Autodesk Fusion 360 part; units mm, degrees
(part 3 of 3)
sketch "Sketch8" plane through (0, 0, 14) normal (0, 0, -1) x (1, 0, 0)
  line L0 (65.5351, 21) -> (80.5351, 21)
  line L1 (80.5351, 21) -> (80.5351, 35)
  line L2 (80.5351, 35) -> (65.5351, 35)
  line L3 (65.5351, 35) -> (65.5351, 21)
  line L4 (80.5351, 21) -> (65.5351, 21)
  line L5 (65.5351, 21) -> (65.5351, 7)
  line L6 (65.5351, 7) -> (80.5351, 7)
  line L7 (80.5351, 7) -> (80.5351, 21)
  line L8 (76.5351, 8) -> (69.5351, 8)
  line L9 (69.5351, 8) -> (69.5351, 34)
  line L10 (69.5351, 34) -> (76.5351, 34)
  line L11 (76.5351, 34) -> (76.5351, 8)
  line L12 (76.5351, 8) -> (69.5351, 34) construction
  line L13 (69.5351, 8) -> (76.5351, 34) construction
  line L14 (80.6351, 20.9) -> (80.6351, 35.1)
  line L15 (80.6351, 35.1) -> (65.4351, 35.1)
  line L16 (65.4351, 35.1) -> (65.4351, 20.9)
  line L17 (65.4351, 20.9) -> (80.6351, 20.9)
  line L18 (80.6351, 6.9) -> (80.6351, 21.1)
  line L19 (80.6351, 21.1) -> (65.4351, 21.1)
  line L20 (65.4351, 21.1) -> (65.4351, 6.9)
  line L21 (65.4351, 6.9) -> (80.6351, 6.9)
  line L22 (81.5351, 20) -> (81.5351, 36)
  line L23 (81.5351, 36) -> (64.5351, 36)
  line L24 (64.5351, 36) -> (64.5351, 20)
  line L25 (81.5351, 6) -> (81.5351, 22)
  line L26 (64.5351, 22) -> (64.5351, 6)
  line L27 (64.5351, 6) -> (81.5351, 6)
  line L28 (65.4351, 20) -> (65.5351, 20)
  line L29 (80.5351, 20) -> (80.6351, 20)
  line L30 (80.6351, 22) -> (80.5351, 22)
  line L31 (65.5351, 22) -> (65.4351, 22)
  point P0 (73.0351, 21)
  dimension "d278" = 7
  dimension "d279" = 26
  dimension "d280" = 0.1
  dimension "d281" = 0.1
  constraint horizontal L8
  constraint perpendicular L8 L9
  constraint parallel L8 L10
  constraint parallel L9 L11
  constraint coincident L12 P0
  constraint coincident L13 P0
  constraint midpoint L0 P0
  constraint coincident L5 L28.end
  constraint coincident L7 L29.start
  constraint coincident L18 L29.end
  constraint coincident L20 L28.start
  constraint coincident L16 L31.end
  constraint coincident L14 L30.start
  constraint coincident L1 L30.end
  constraint collinear L30 L31
  constraint coincident L3 L31.start
  measures "d278" distance of L9.end L10.end
  measures "d279" distance of L8.end L9.end
extrude "Extrude41" add sketch "Sketch8" against normal blind 8.5 from surface at 12 contours L0 L4 L9 L11 L19 | L0 L4 L9 L11 L17 | L8 L9 L11 L17 | L9 L10 L11 L19 bodies 13
fillet "Fillet7" radius 1.5 4 edges at (76.5351, -21, 10.5) (69.5351, -21, 10.5) (73.0351, -34, 10.5) (73.0351, -8, 10.5) on bodies 13
extrude "Extrude42" cut sketch "Sketch8" against normal blind 4 contours L0 L3 L4 L9 L19 | L3 L5 L16 L17 L19 L20 | L0 L4 L5 L9 L17 | L3 L16 L19 L31 | L1 L2 L3 L9 L10 L11 L19 | L5 L6 L7 L8 L9 L11 L17 | L5 L17 L20 L28 | L0 L1 L4 L11 L19 | L0 L4 L7 L11 L17 | L1 L2 L3 L14 L15 L16 L30 L31 | L5 L6 L7 L18 L20 L21 L28 L29 | L1 L7 L14 L17 L18 L19 | L1 L14 L19 L30 | L7 L17 L18 L29 | L22 L23 L24 L25 L26 L27 bodies 15
extrude "Extrude43" cut sketch "Sketch8" against normal blind 6 contours L0 L3 L4 L9 L19 | L0 L4 L5 L9 L17 | L1 L2 L3 L9 L10 L11 L19 | L5 L6 L7 L8 L9 L11 L17 | L0 L1 L4 L11 L19 | L0 L4 L7 L11 L17 bodies 12
sketch "Sketch9" plane through (0, 0, 10.5) normal (0, 0, 1) x (-1, 0, 0)
  line L0 (-71.0351, 9.5) -> (-71.0351, 32.5)
  line L1 (-71.0351, 32.5) -> (-75.0351, 32.5)
  line L2 (-75.0351, 32.5) -> (-75.0351, 9.5)
  line L3 (-75.0351, 9.5) -> (-71.0351, 9.5)
  line L4 (-71.0351, 20) -> (-75.0351, 20)
  line L5 (-75.0351, 20) -> (-75.0351, 22.4)
  line L6 (-75.0351, 22.4) -> (-71.0351, 22.4)
  line L7 (-71.0351, 22.4) -> (-71.0351, 20)
  line L8 (-75.0351, 20) -> (-71.0351, 20) construction
  line L9 (-71.0351, 20) -> (-71.0351, 12.1) construction
  line L10 (-71.0351, 12.1) -> (-75.0351, 12.1) construction
  line L11 (-75.0351, 12.1) -> (-75.0351, 20) construction
  line L12 (-75.0351, 22.4) -> (-71.0351, 22.4) construction
  line L13 (-71.0351, 22.4) -> (-71.0351, 30.3) construction
  line L14 (-71.0351, 30.3) -> (-75.0351, 30.3) construction
  line L15 (-75.0351, 30.3) -> (-75.0351, 22.4) construction
  line L16 (-75.0351, 30.3) -> (-71.0351, 30.3)
  line L17 (-71.0351, 30.3) -> (-71.0351, 32.3)
  line L18 (-71.0351, 32.3) -> (-75.0351, 32.3)
  line L19 (-75.0351, 32.3) -> (-75.0351, 30.3)
  line L20 (-75.0351, 12.1) -> (-71.0351, 12.1)
  line L21 (-71.0351, 12.1) -> (-71.0351, 10.1)
  line L22 (-71.0351, 10.1) -> (-75.0351, 10.1)
  line L23 (-75.0351, 10.1) -> (-75.0351, 12.1)
  dimension "d295" = 2.4
  dimension "d296" = 7.9
  dimension "d297" = 7.9
  dimension "d298" = 2
  dimension "d299" = 2
  constraint horizontal L4
  constraint perpendicular L4 L5
  constraint parallel L4 L6
  constraint parallel L5 L7
  constraint horizontal L8
  constraint vertical L9
  constraint horizontal L10
  constraint vertical L11
  constraint horizontal L12
  constraint vertical L13
  constraint horizontal L14
  constraint vertical L15
  constraint horizontal L16
  constraint vertical L17
  constraint horizontal L18
  constraint vertical L19
  constraint horizontal L20
  constraint vertical L21
  constraint horizontal L22
  constraint vertical L23
  measures "d295" distance of L4.end L5.end
  measures "d296" distance of L4.end L10.end
  measures "d297" distance of L5.end L14.end
  measures "d298" distance of L14.end L18.end
  measures "d299" distance of L10.end L22.end
extrude "Extrude44" add sketch "Sketch9" along normal blind 2.6 contours L0 L2 L20 L21 L22 L23 | L0 L2 L4 L5 L6 L7 | L0 L2 L16 L17 L18 L19 bodies 13
chamfer "Chamfer9" distance 1 angle 45 6 edges at (53.5294, -9.8942, 12.5) (24.8248, -9.8942, 12.5) (1.062, -9.8942, 12.5) (24.8248, -32.8942, 12.5) (42.3772, -32.8942, 12.5) (1.062, -32.8942, 12.5) on bodies 12
extrude "Extrude45" add sketch "Sketch7" along normal blind 2 from surface at 7 contours L55 L69 L73 L86 | L68 L69 L70 L73 L74 L75 L87 L88 | L55 L68 L75 L84 L85 bodies 16
sketch "Sketch10" plane through (0, 0, 0) normal (0, 0, 1) x (1, 0, 0)
  line L0 (0, -124.6556) -> (3.5, -124.6556)
  line L1 (3.5, -124.6556) -> (3.5, -128.1556)
  line L2 (3.5, -128.1556) -> (0, -128.1556)
  line L3 (0, -128.1556) -> (0, -124.6556)
  line L4 (-1, -129.1556) -> (-1, -123.6556)
  line L5 (-1, -123.6556) -> (4.5, -123.6556)
  line L6 (4.5, -123.6556) -> (4.5, -129.1556)
  line L7 (4.5, -129.1556) -> (-1, -129.1556)
  line L8 (19.9601, -130.9847) -> (33.4601, -130.9847)
  line L9 (33.4601, -130.9847) -> (33.4601, -103.5847)
  line L10 (33.4601, -103.5847) -> (19.9601, -103.5847)
  line L11 (19.9601, -103.5847) -> (19.9601, -130.9847)
  line L12 (26.7101, -130.9847) -> (26.7101, -123.1847) construction
  line L13 (19.9601, -123.1847) -> (26.5601, -123.1847) construction
  line L14 (30.4601, -119.2847) -> (22.6601, -119.2847) construction
  line L15 (22.6601, -119.2847) -> (22.6601, -127.0847) construction
  line L16 (22.6601, -127.0847) -> (30.4601, -127.0847) construction
  line L17 (30.4601, -127.0847) -> (30.4601, -119.2847) construction
  line L18 (30.4601, -119.2847) -> (22.6601, -127.0847) construction
  line L19 (22.6601, -119.2847) -> (30.4601, -127.0847) construction
  line L20 (19.9601, -130.9847) -> (22.4601, -130.9847)
  line L21 (22.4601, -130.9847) -> (22.4601, -119.2847)
  line L22 (22.4601, -119.2847) -> (19.9601, -119.2847)
  line L23 (19.9601, -119.2847) -> (19.9601, -130.9847)
  line L24 (33.4601, -130.9847) -> (30.8601, -130.9847)
  line L25 (30.8601, -130.9847) -> (30.8601, -119.2847)
  line L26 (30.8601, -119.2847) -> (33.4601, -119.2847)
  line L27 (33.4601, -119.2847) -> (33.4601, -130.9847)
  line L28 (28.2101, -127.778) -> (25.2101, -127.778)
  line L29 (25.2101, -127.778) -> (25.2101, -129.778)
  line L30 (25.2101, -129.778) -> (28.2101, -129.778)
  line L31 (28.2101, -129.778) -> (28.2101, -127.778)
  line L32 (28.2101, -127.778) -> (25.2101, -129.778) construction
  line L33 (25.2101, -127.778) -> (28.2101, -129.778) construction
  line L34 (25.2101, -129.778) -> (25.2101, -130.9847)
  line L35 (28.2101, -129.778) -> (28.2101, -130.9847)
  point P0 (26.5601, -123.1847)
  point P1 (26.7101, -128.778)
  dimension "d307" = 3.5
  dimension "d308" = 3.5
  dimension "d309" = -1
  dimension "d314" = 13.5
  dimension "d315" = 27.4
  dimension "d316" = 7.8
  dimension "d317" = 6.6
  dimension "d318" = 7.8
  dimension "d319" = 7.8
  dimension "d320" = 2.5
  dimension "d321" = 2.6
  dimension "d322" = 3
  dimension "d323" = 2
  constraint horizontal L0
  constraint vertical L1
  constraint horizontal L2
  constraint vertical L3
  constraint horizontal L8
  constraint vertical L9
  constraint horizontal L10
  constraint vertical L11
  constraint midpoint L8 L12.start
  constraint perpendicular L8 L12
  constraint coincident L11 L13.start
  constraint perpendicular L12 L13
  constraint horizontal L14
  constraint perpendicular L14 L15
  constraint parallel L14 L16
  constraint parallel L15 L17
  constraint coincident L18 P0
  constraint coincident L19 P0
  constraint coincident P0 L13.end
  constraint horizontal L20
  constraint vertical L21
  constraint horizontal L22
  constraint vertical L23
  constraint horizontal L24
  constraint vertical L25
  constraint horizontal L26
  constraint vertical L27
  constraint horizontal L28
  constraint perpendicular L28 L29
  constraint parallel L28 L30
  constraint parallel L29 L31
  constraint coincident L32 P1
  constraint coincident L33 P1
  constraint coincident L12 P1
  constraint coincident L8 L34.end
  constraint perpendicular L8 L34
  constraint coincident L8 L35.end
  constraint perpendicular L8 L35
  measures "d307" distance of L0.start L0.end
  measures "d308" distance of L0.start L2.end
  measures "d314" distance of L8.start L8.end
  measures "d315" distance of L8.start L10.end
  measures "d316" distance of L12.start L12.end
  measures "d317" distance of L13.start P0
  measures "d318" distance of L15.end L16.end
  measures "d319" distance of L14.end L15.end
  measures "d320" distance of L8.start L20.end
  measures "d321" distance of L8.end L24.end
  measures "d322" distance of L29.end L30.end
  measures "d323" distance of L28.end L29.end
extrude "Extrude46" add sketch "Sketch10" along normal blind 7.3 separate body contours L0 L1 L2 L3 makes body 19
extrude "Extrude47" add sketch "Sketch10" along normal blind 1 contours L4 L5 L6 L7 bodies 19
extrude "Extrude48" add sketch "Sketch10" against normal blind 2 separate body contours L8 L11 L20 L21 L22 L23 | L8 L9 L10 L11 L21 L22 L25 L26 L28 L29 L31 L34 L35 | L8 L30 L34 L35 | L28 L29 L30 L31 | L8 L9 L24 L25 L26 L27 makes body 20
sketch "Sketch11" plane through (0, 0, 16.5) normal (0, 0, 1) x (-1, 0, 0)
  line L0 (-80.5351, 35) -> (-65.5351, 35)
  line L1 (-65.5351, 35) -> (-65.5351, 7)
  line L2 (-65.5351, 7) -> (-80.5351, 7)
  line L3 (-80.5351, 7) -> (-80.5351, 35)
  line L4 (2, -114) -> (3, -114)
  line L5 (3, -114) -> (3, -129)
  line L6 (3, -129) -> (15, -129)
  line L7 (15, -129) -> (15, -114)
  line L8 (15, -114) -> (16, -114)
  line L9 (16, -114) -> (16, 35)
  arc A0 (16, 35) -> (6, 45) centre (6, 35) ccw
  line L10 (6, 45) -> (-84, 45)
  arc A1 (-84, 45) -> (-94, 35) centre (-84, 35) ccw
  line L11 (-94, 35) -> (-94, -114)
  line L12 (-94, -114) -> (-93, -114)
  line L13 (-93, -114) -> (-93, -129)
  line L14 (-93, -129) -> (-81, -129)
  line L15 (-81, -129) -> (-81, -114)
  line L16 (-81, -114) -> (-80, -114)
  line L17 (-80, -114) -> (-80, -89.1708)
  line L18 (-80, -89.1708) -> (-78, -89.1708)
  line L19 (-78, -89.1708) -> (-78, -10)
  arc A2 (-68, 0) -> (-78, -10) centre (-68, -10) ccw
  line L20 (-68, 0) -> (-46.5, 0)
  arc A3 (0, -10) -> (-10, 0) centre (-10, -10) ccw
  line L21 (0, -10) -> (0, -89.1708)
  line L22 (0, -89.1708) -> (2, -89.1708)
  line L23 (2, -89.1708) -> (2, -114)
  circle A4 centre (8.0138, 36.9996) radius 2.75
  circle A5 centre (8.0138, -80.0004) radius 2.75
  circle A6 centre (-85.9862, -80.0004) radius 2.75
  circle A7 centre (-85.9862, 36.9996) radius 2.75
  line L24 (-58, 26.0298) -> (-57, 26.0298)
  line L25 (-57, 26.0298) -> (-57, 34.3942)
  line L26 (-57, 34.3942) -> (2.5, 34.3942)
  line L27 (2.5, 34.3942) -> (2.5, 26.0298)
  line L28 (2.5, 26.0298) -> (3.5, 26.0298)
  line L29 (3.5, 26.0298) -> (3.5, 12.982)
  line L30 (3.5, 12.982) -> (2.5, 12.982)
  line L31 (2.5, 12.982) -> (2.5, 8.3942)
  line L32 (2.5, 8.3942) -> (-57, 8.3942)
  line L33 (-57, 8.3942) -> (-57, 12.982)
  line L34 (-57, 12.982) -> (-58, 12.982)
  line L35 (-58, 12.982) -> (-58, 26.0298)
  line L36 (-79.2351, 8.3) -> (-79.2351, 20.7)
  line L37 (-79.2351, 20.7) -> (-66.8351, 20.7)
  line L38 (-66.8351, 20.7) -> (-66.8351, 8.3)
  line L39 (-66.8351, 8.3) -> (-79.2351, 8.3)
  line L40 (-65.5351, 21) -> (-80.5351, 21)
  line L41 (-80.5351, 21) -> (-80.5351, 7)
  line L42 (-80.5351, 7) -> (-65.5351, 7)
  line L43 (-65.5351, 7) -> (-65.5351, 21)
  line L44 (-79.2351, 33.7) -> (-66.8351, 33.7)
  line L45 (-66.8351, 33.7) -> (-66.8351, 21.3)
  line L46 (-66.8351, 21.3) -> (-79.2351, 21.3)
  line L47 (-79.2351, 21.3) -> (-79.2351, 33.7)
  line L48 (-80.5351, 21) -> (-65.5351, 21)
  line L49 (-65.5351, 21) -> (-65.5351, 35)
  line L50 (-65.5351, 35) -> (-80.5351, 35)
  line L51 (-80.5351, 35) -> (-80.5351, 21)
  line L52 (-81.3351, 21.8) -> (-81.3351, 6.2)
  line L53 (-81.3351, 6.2) -> (-64.7351, 6.2)
  line L54 (-64.7351, 6.2) -> (-64.7351, 21.8)
  line L55 (-64.7351, 21.8) -> (-81.3351, 21.8)
  line L56 (-81.3351, 6.2) -> (-81.3351, 35.8)
  line L57 (-81.3351, 35.8) -> (-64.7351, 35.8)
  line L58 (-64.7351, 35.8) -> (-64.7351, 6.2)
  line L59 (-64.7351, 6.2) -> (-81.3351, 6.2)
  line L60 (-46.5, 0) -> (-46.5, 4)
  line L61 (-46.5, 4) -> (-31.5, 4)
  line L62 (-31.5, 4) -> (-31.5, 0)
  line L63 (-31.5, 0) -> (-10, 0)
  dimension "d332" = 0.8
  dimension "d333" = -0.8
extrude "Extrude51" cut sketch "Sketch11" against normal blind 3 contours L0 L1 L3 L49 L50 L51 L55 L56 L57 L58 | L1 L2 L3 L41 L42 L43 L49 L51 L52 L53 L54 L55 L56 L58 L59 bodies 12
sketch "Sketch12" plane through (0, 0, 20) normal (0, 0, 1) x (-1, 0, 0)
  line L0 (3, -114) -> (15, -114)
  line L1 (15, -114) -> (15, 35)
  arc A0 (15, 35) -> (6, 44) centre (6, 35) ccw
  line L2 (6, 44) -> (-84, 44)
  arc A1 (-84, 44) -> (-93, 35) centre (-84, 35) ccw
  line L3 (-93, 35) -> (-93, -114)
  line L4 (-93, -114) -> (-81, -114)
  line L5 (-81, -114) -> (-81, -10)
  arc A2 (-68, 3) -> (-81, -10) centre (-68, -10) ccw
  line L6 (-68, 3) -> (-10, 3)
  arc A3 (3, -10) -> (-10, 3) centre (-10, -10) ccw
  line L7 (3, -10) -> (3, -114)
  circle A4 centre (8.0138, -80.0004) radius 3.6
  circle A5 centre (-85.9862, 36.9996) radius 3.6
  circle A6 centre (-85.9862, -80.0004) radius 3.6
  circle A7 centre (8.0138, 36.9996) radius 3.6
  line L8 (3.5, 7.3942) -> (-58, 7.3942)
  line L9 (-58, 7.3942) -> (-58, 35.3942)
  line L10 (-58, 35.3942) -> (3.5, 35.3942)
  line L11 (3.5, 35.3942) -> (3.5, 7.3942)
  line L12 (-79.5351, 34) -> (-66.5351, 34)
  line L13 (-66.5351, 34) -> (-66.5351, 8)
  line L14 (-66.5351, 8) -> (-79.5351, 8)
  line L15 (-79.5351, 8) -> (-79.5351, 34)
  line L16 (-58, 35.3942) -> (3.5, 35.3942)
  line L17 (3.5, 35.3942) -> (3.5, 27.3942)
  line L18 (-0.5, 27.3942) -> (-44, 27.3942)
  line L19 (-58, 27.3942) -> (-58, 35.3942)
  line L20 (3.5, 27.3942) -> (0.5, 27.3942)
  line L21 (0.5, 26.3942) -> (0.5, 14.8942)
  line L22 (0.5, 7.3942) -> (3.5, 7.3942)
  line L23 (3.5, 7.3942) -> (3.5, 27.3942)
  line L24 (-58, 27.3942) -> (-45, 27.3942)
  line L25 (-45, 26.3942) -> (-45, 14.8942)
  line L26 (-45, 7.3942) -> (-58, 7.3942)
  line L27 (-58, 7.3942) -> (-58, 27.3942)
  line L28 (0.5, 7.3942) -> (-45, 7.3942)
  line L29 (-45, 7.3942) -> (-45, 13.8942)
  line L30 (-44, 13.8942) -> (-0.5, 13.8942)
  line L31 (0.5, 13.8942) -> (0.5, 7.3942)
  arc A8 (-0.5, 13.8942) -> (0.5, 14.8942) centre (-0.5, 14.8942) ccw
  arc A9 (0.5, 26.3942) -> (-0.5, 27.3942) centre (-0.5, 26.3942) ccw
  arc A10 (-44, 27.3942) -> (-45, 26.3942) centre (-44, 26.3942) ccw
  arc A11 (-45, 14.8942) -> (-44, 13.8942) centre (-44, 14.8942) ccw
  dimension "d336" = 8
  dimension "d337" = 3
  dimension "d338" = 13
  dimension "d339" = 6.5
  dimension "d420" = 1
  constraint horizontal L16
  constraint vertical L17
  constraint horizontal L18
  constraint vertical L19
  constraint coincident L9.end L10.start
  constraint horizontal L20
  constraint vertical L21
  constraint horizontal L22
  constraint vertical L23
  constraint horizontal L24
  constraint vertical L25
  constraint horizontal L26
  constraint vertical L27
  constraint horizontal L28
  constraint vertical L29
  constraint horizontal L30
  constraint vertical L31
  constraint coincident L31.start L30
  constraint coincident L22.start L21
  constraint tangent L30 A8
  constraint tangent L21 A8
  constraint coincident L20.end L21
  constraint coincident L17.end L18
  constraint tangent L21 A9
  constraint tangent L18 A9
  constraint equal A8 A9
  constraint coincident L19.start L18
  constraint coincident L24.end L25
  constraint tangent L18 A10
  constraint tangent L25 A10
  constraint equal A8 A10
  constraint coincident L29.end L30
  constraint coincident L26.start L25
  constraint tangent L30 A11
  constraint tangent L25 A11
  constraint equal A8 A11
  measures "d336" distance of L9.end L19.start
  measures "d337" distance of L17.end L20.end
  measures "d338" distance of L19.start L24.end
  measures "d339" distance of L22.start L31.start
  measures "d420" radius of A8
extrude "Extrude52" add sketch "Sketch12" against normal blind 0.4 contours L8 L9 L10 L11 L16 L17 L19 L22 L23 L26 L27 L28 bodies 15
extrude "Extrude49" add sketch "Sketch10" against normal blind 4 contours L8 L11 L20 L21 L22 L23 | L8 L30 L34 L35 | L28 L29 L30 L31 | L8 L9 L24 L25 L26 L27 bodies 20
sketch "Sketch13" plane through (46.5, 0, 0) normal (-1, 0, 0) x (0, -1, 0)
  line L0 (0, 2) -> (4, 2)
  line L1 (4, 2) -> (4, 16)
  line L2 (0, 16.5) -> (0, 2)
  line L3 (0, 2) -> (1, 2)
  line L4 (1, 2) -> (1, 14)
  line L5 (0, 14) -> (0, 2)
  line L6 (4, 2) -> (3, 2)
  line L7 (3, 2) -> (3, 14)
  line L8 (4, 14) -> (4, 2)
  line L9 (4, 16.5) -> (0, 16.5)
  line L10 (4, 16) -> (4, 16.5)
  line L11 (4, 14) -> (4, 16.5)
  line L12 (4, 16.5) -> (3, 16.5)
  line L13 (3, 16.5) -> (3, 14)
  line L14 (0, 14) -> (0, 16.5)
  line L15 (0, 16.5) -> (1, 16.5)
  line L16 (1, 16.5) -> (1, 14)
  dimension "d342" = 1
  dimension "d343" = 1
  constraint horizontal L3
  constraint vertical L4
  constraint vertical L5
  constraint coincident L0.start L2.end
  constraint horizontal L6
  constraint vertical L7
  constraint vertical L8
  constraint coincident L0.end L1.start
  constraint vertical L11
  constraint horizontal L12
  constraint vertical L13
  constraint coincident L9.start L10.end
  constraint vertical L14
  constraint horizontal L15
  constraint vertical L16
  constraint coincident L2.start L9.end
  measures "d342" distance of L0.start L3.end
  measures "d343" distance of L0.end L6.end
extrude "Extrude53" add sketch "Sketch13" along normal blind 1.5 contours L0 L2 L3 L4 L5 L9 L14 L15 L16 | L0 L1 L6 L7 L8 L9 L10 L11 L12 L13 bodies 12
extrude "Extrude54" add sketch "Sketch13" against normal blind 1.5 from surface at 15 contours L0 L2 L3 L4 L5 L9 L14 L15 L16 | L0 L1 L6 L7 L8 L9 L10 L11 L12 L13 bodies 12
sketch "Sketch14" plane through (0, 0, 16.5) normal (0, 0, -1) x (1, 0, 0)
  line L0 (33, 4) -> (33, 3)
  line L1 (33, 3) -> (31.5, 3)
  line L2 (31.5, 3) -> (31.5, 1)
  line L3 (31.5, 1) -> (33, 1)
  line L4 (33, 1) -> (33, 0)
  line L5 (33, 0) -> (45, 0)
  line L6 (45, 0) -> (45, 1)
  line L7 (45, 1) -> (46.5, 1)
  line L8 (46.5, 1) -> (46.5, 3)
  line L9 (46.5, 3) -> (45, 3)
  line L10 (45, 3) -> (45, 4)
  line L11 (45, 4) -> (33, 4)
  line L12 (44.9, 1.1) -> (46.4, 1.1)
  line L13 (46.4, 1.1) -> (46.4, 2.9)
  line L14 (46.4, 2.9) -> (44.9, 2.9)
  line L15 (44.9, 2.9) -> (44.9, 3.9)
  line L16 (44.9, 3.9) -> (33.1, 3.9)
  line L17 (33.1, 3.9) -> (33.1, 2.9)
  line L18 (33.1, 2.9) -> (31.6, 2.9)
  line L19 (31.6, 2.9) -> (31.6, 1.1)
  line L20 (31.6, 1.1) -> (33.1, 1.1)
  line L21 (33.1, 1.1) -> (33.1, 0.1)
  line L22 (44.9, 0.1) -> (44.9, 1.1)
  line L23 (44.9, 0.1) -> (44.9, 0)
  line L24 (33.1, 0.1) -> (33.1, 0)
  line L25 (81.3351, 35.8) -> (64.7351, 35.8)
  line L26 (64.7351, 35.8) -> (64.7351, 6.2)
  line L27 (64.7351, 6.2) -> (81.3351, 6.2)
  line L28 (81.3351, 6.2) -> (81.3351, 35.8)
  line L29 (-2, -114) -> (-3, -114)
  line L30 (-3, -114) -> (-3, -129)
  line L31 (-3, -129) -> (-15, -129)
  line L32 (-15, -129) -> (-15, -114)
  line L33 (-15, -114) -> (-16, -114)
  line L34 (-16, -114) -> (-16, 35)
  arc A0 (-6, 45) -> (-16, 35) centre (-6, 35) ccw
  line L35 (-6, 45) -> (84, 45)
  arc A1 (94, 35) -> (84, 45) centre (84, 35) ccw
  line L36 (94, 35) -> (94, -114)
  line L37 (94, -114) -> (93, -114)
  line L38 (93, -114) -> (93, -129)
  line L39 (93, -129) -> (81, -129)
  line L40 (81, -129) -> (81, -114)
  line L41 (81, -114) -> (80, -114)
  line L42 (80, -114) -> (80, -89.1708)
  line L43 (80, -89.1708) -> (78, -89.1708)
  line L44 (78, -89.1708) -> (78, -10)
  arc A2 (78, -10) -> (68, 0) centre (68, -10) ccw
  line L45 (68, 0) -> (45, 0)
  line L46 (45, 0) -> (45, 1)
  line L47 (45, 1) -> (46.5, 1)
  line L48 (46.5, 1) -> (46.5, 3)
  line L49 (46.5, 3) -> (45, 3)
  line L50 (45, 3) -> (45, 4)
  line L51 (45, 4) -> (33, 4)
  line L52 (33, 4) -> (33, 3)
  line L53 (33, 3) -> (31.5, 3)
  line L54 (31.5, 3) -> (31.5, 1)
  line L55 (31.5, 1) -> (33, 1)
  line L56 (33, 1) -> (33, 0)
  line L57 (33, 0) -> (10, 0)
  arc A3 (10, 0) -> (0, -10) centre (10, -10) ccw
  line L58 (0, -10) -> (0, -89.1708)
  line L59 (0, -89.1708) -> (-2, -89.1708)
  line L60 (-2, -89.1708) -> (-2, -114)
  circle A4 centre (-8.0138, 36.9996) radius 2.75
  circle A5 centre (-8.0138, -80.0004) radius 2.75
  circle A6 centre (85.9862, -80.0004) radius 2.75
  circle A7 centre (85.9862, 36.9996) radius 2.75
  line L61 (58, 26.0298) -> (57, 26.0298)
  line L62 (57, 26.0298) -> (57, 34.3942)
  line L63 (57, 34.3942) -> (-2.5, 34.3942)
  line L64 (-2.5, 34.3942) -> (-2.5, 26.0298)
  line L65 (-2.5, 26.0298) -> (-3.5, 26.0298)
  line L66 (-3.5, 26.0298) -> (-3.5, 12.982)
  line L67 (-3.5, 12.982) -> (-2.5, 12.982)
  line L68 (-2.5, 12.982) -> (-2.5, 8.3942)
  line L69 (-2.5, 8.3942) -> (57, 8.3942)
  line L70 (57, 8.3942) -> (57, 12.982)
  line L71 (57, 12.982) -> (58, 12.982)
  line L72 (58, 12.982) -> (58, 26.0298)
  constraint coincident L5 L23.end
  constraint perpendicular L5 L23
  constraint coincident L5 L24.end
  constraint perpendicular L5 L24
extrude "Extrude55" add sketch "Sketch14" along normal blind 14.5 separate body contours L5 L12 L13 L14 L15 L16 L17 L18 L19 L20 L21 L22 L23 L24 makes body 21
sketch "Sketch15" plane through (0, 0, 0) normal (0, 1, 0) x (-1, 0, 0)
  line L0 (-33.1, 16.5) -> (-44.9, 16.5)
  line L1 (-44.9, 16.5) -> (-44.9, 2)
  line L2 (-44.9, 2) -> (-33.1, 2)
  line L3 (-33.1, 2) -> (-33.1, 16.5)
  line L4 (-7.5, 8) -> (-70.5, 8)
  arc A0 (-70.5, 8) -> (-73, 5.5) centre (-70.5, 5.5) ccw
  line L5 (-73, 5.5) -> (-5, 5.5)
  arc A1 (-5, 5.5) -> (-7.5, 8) centre (-7.5, 5.5) ccw
  line L6 (-5, 5.5) -> (-73, 5.5)
  line L7 (-73, 5.5) -> (-73, 2)
  line L8 (-73, 2) -> (-5, 2)
  line L9 (-5, 2) -> (-5, 5.5)
  line L10 (-39, 8) -> (-39, 16.5) construction
  line L11 (-39, 8) -> (-39, 10) construction
  line L12 (-39, 10) -> (-33.1, 10) construction
  line L13 (-39, 10) -> (-44.9, 10) construction
  line L14 (-39, 10) -> (-39, 13) construction
  line L15 (-35.8, 10) -> (-42.2, 10)
  line L16 (-43.5, 11.3) -> (-43.5, 11.7)
  line L17 (-42.2, 13) -> (-35.8, 13)
  line L18 (-34.5, 11.7) -> (-34.5, 11.3)
  line L19 (-34.5, 10) -> (-43.5, 13) construction
  line L20 (-43.5, 10) -> (-34.5, 13) construction
  arc A2 (-42.2, 13) -> (-43.5, 11.7) centre (-42.2, 11.7) ccw
  arc A3 (-43.5, 11.3) -> (-42.2, 10) centre (-42.2, 11.3) ccw
  arc A4 (-35.8, 10) -> (-34.5, 11.3) centre (-35.8, 11.3) ccw
  arc A5 (-34.5, 11.7) -> (-35.8, 13) centre (-35.8, 11.7) ccw
  arc A6 (-34.8, 11.7) -> (-35.8, 12.7) centre (-35.8, 11.7) ccw
  line L21 (-42.2, 12.7) -> (-35.8, 12.7)
  arc A7 (-42.2, 12.7) -> (-43.2, 11.7) centre (-42.2, 11.7) ccw
  line L22 (-43.2, 11.3) -> (-43.2, 11.7)
  arc A8 (-43.2, 11.3) -> (-42.2, 10.3) centre (-42.2, 11.3) ccw
  line L23 (-35.8, 10.3) -> (-42.2, 10.3)
  arc A9 (-35.8, 10.3) -> (-34.8, 11.3) centre (-35.8, 11.3) ccw
  line L24 (-34.8, 11.7) -> (-34.8, 11.3)
  line L25 (-43.2, 11.5) -> (-43.5, 11.5) construction
  line L26 (-34.8, 11.5) -> (-34.5, 11.5) construction
  line L27 (-34.8, 11) -> (-34.5351, 11)
  line L28 (-34.8, 12) -> (-34.5351, 12)
  line L29 (-34.5351, 12) -> (-34.8461, 12)
  line L30 (-34.5351, 11) -> (-34.8461, 11)
  line L31 (-43.2, 12) -> (-43.5, 12)
  line L32 (-43.1539, 12) -> (-43.4649, 12)
  line L33 (-43.1539, 11) -> (-43.4649, 11)
  point P0 (-39, 11.5)
  dimension "d399" = 2
  dimension "d400" = 3
  dimension "d401" = 9
  dimension "d402" = 3
  dimension "d403" = 1.3
  dimension "d404" = 0.3
  dimension "d414" = 0.5
  constraint midpoint L4 L10.start
  constraint midpoint L0 L10.end
  constraint perpendicular L4 L11
  constraint coincident L3 L12.end
  constraint perpendicular L3 L12
  constraint coincident L1 L13.end
  constraint perpendicular L1 L13
  constraint perpendicular L12 L14
  constraint horizontal L15
  constraint perpendicular L15 L16
  constraint parallel L15 L17
  constraint parallel L16 L18
  constraint coincident L19 P0
  constraint coincident L20 P0
  constraint midpoint L14 P0
  constraint coincident L19.end L17
  constraint coincident L19.end L16
  constraint tangent L17 A2
  constraint tangent L16 A2
  constraint coincident L20.start L16
  constraint coincident L20.start L15
  constraint tangent L16 A3
  constraint tangent L15 A3
  constraint equal A2 A3
  constraint coincident L19.start L15
  constraint coincident L19.start L18
  constraint tangent L15 A4
  constraint tangent L18 A4
  constraint equal A2 A4
  constraint coincident L20.end L18
  constraint coincident L20.end L17
  constraint tangent L18 A5
  constraint tangent L17 A5
  constraint equal A2 A5
  constraint midpoint L22 L25.start
  constraint midpoint L16 L25.end
  constraint perpendicular L16 L25
  constraint midpoint L24 L26.start
  constraint midpoint L18 L26.end
  constraint perpendicular L18 L26
  constraint parallel L28 L29
  constraint parallel L27 L30
  constraint coincident A6 L29.end
  constraint coincident A9 L30.end
  constraint coincident A4 L27.end
  constraint coincident A5 L28.end
  constraint coincident A7 L32.start
  constraint coincident A2 L32.end
  constraint coincident L31 L32.end
  constraint parallel L31 L32
  constraint coincident A8 L33.start
  constraint coincident A3 L33.end
  constraint parallel L32 L33
  measures "d399" distance of L10.start L11.end
  measures "d400" distance of L11.end L14.end
  measures "d401" distance of L19.end L20.end
  measures "d402" distance of L20.start L19.end
  measures "d403" radius of A2
sketch "Sketch17" plane through (0, -3.9, 0) normal (0, -1, 0) x (1, 0, 0)
  line L0 (44.9, 16.5) -> (33.1, 16.5)
  line L1 (33.1, 16.5) -> (33.1, 2)
  line L2 (33.1, 2) -> (44.9, 2)
  line L3 (44.9, 2) -> (44.9, 16.5)
  line L4 (33.1, 7.1786) -> (44.9, 7.1786)
  line L5 (44.9, 7.1786) -> (44.9, 15.0576)
  line L6 (44.9, 15.0576) -> (33.1, 15.0576)
  line L7 (33.1, 15.0576) -> (33.1, 7.1786)
  constraint horizontal L4
  constraint vertical L5
  constraint horizontal L6
  constraint vertical L7
  constraint coincident L3 L5.end
  constraint coincident L1 L4.start
extrude "Extrude65" add sketch "Sketch17" along normal blind 2 contours L1 L3 L4 L5 L6 L7 bodies 21
extrude "Extrude66" cut sketch "Sketch15" against normal blind 7.6 contours A6 L21 A7 L22 A8 L23 A9 L24 bodies 21
extrude "Extrude67" cut sketch "Sketch15" against normal blind 2.5 from surface at -1 contours L15 A3 A4 A8 L23 A9 L27 L30 L33 | L18 A4 A5 A6 A9 L24 L27 L28 L29 L30 | L16 A2 A3 A7 L22 A8 L31 L32 L33 | L17 A2 A5 A6 L21 A7 L28 L29 L31 L32 bodies 21
extrude "Extrude68" cut sketch "Sketch15" against normal blind 9.1 from surface at -3 contours L18 A4 A5 A6 A9 L24 L27 L28 L29 L30 | L16 A2 A3 A7 L22 A8 L31 L32 L33 bodies 21
ref_plane "WorkPlane6" through (39, -2.95, 11.5) normal (0, 0, 1) x (-1, 0, 0)
split "Split8" by plane through (39, -2.95, 11.5) normal (0, 0, 1) bodies 21 makes body 22 at (37.0333, -2.3, 16.5)
chamfer "Chamfer12" distance 2 angle 45 1 edges at (39, -5.9, 7.1786) on bodies 21
chamfer "Chamfer13" distance 2 angle 45 1 edges at (39, -5.9, 15.0576) on bodies 22
sketch "Sketch18" plane through (0, 0, 20) normal (0, 0, 1) x (-1, 0, 0)
  arc A0 (0.5, 26.3942) -> (-0.5, 27.3942) centre (-0.5, 26.3942) ccw
  line L0 (0.5, 26.3942) -> (0.5, 14.8942)
  arc A1 (-0.5, 13.8942) -> (0.5, 14.8942) centre (-0.5, 14.8942) ccw
  line L1 (-0.5, 13.8942) -> (-44, 13.8942)
  arc A2 (-45, 14.8942) -> (-44, 13.8942) centre (-44, 14.8942) ccw
  line L2 (-45, 14.8942) -> (-45, 26.3942)
  arc A3 (-44, 27.3942) -> (-45, 26.3942) centre (-44, 26.3942) ccw
  line L3 (-44, 27.3942) -> (-0.5, 27.3942)
  line L4 (3, -114) -> (15, -114)
  line L5 (15, -114) -> (15, 35)
  arc A4 (15, 35) -> (6, 44) centre (6, 35) ccw
  line L6 (6, 44) -> (-84, 44)
  arc A5 (-84, 44) -> (-93, 35) centre (-84, 35) ccw
  line L7 (-93, 35) -> (-93, -114)
  line L8 (-93, -114) -> (-81, -114)
  line L9 (-81, -114) -> (-81, -10)
  arc A6 (-68, 3) -> (-81, -10) centre (-68, -10) ccw
  line L10 (-68, 3) -> (-10, 3)
  arc A7 (3, -10) -> (-10, 3) centre (-10, -10) ccw
  line L11 (3, -10) -> (3, -114)
  circle A8 centre (8.0138, -80.0004) radius 3.6
  circle A9 centre (-85.9862, 36.9996) radius 3.6
  circle A10 centre (-85.9862, -80.0004) radius 3.6
  circle A11 centre (8.0138, 36.9996) radius 3.6
  line L12 (-79.5351, 34) -> (-66.5351, 34)
  line L13 (-66.5351, 34) -> (-66.5351, 8)
  line L14 (-66.5351, 8) -> (-79.5351, 8)
  line L15 (-79.5351, 8) -> (-79.5351, 34)
  arc A12 (-48, 14.8942) -> (-44, 10.8942) centre (-44, 14.8942) ccw
  line L16 (-0.5, 10.8942) -> (-44, 10.8942)
  arc A13 (-0.5, 10.8942) -> (3.5, 14.8942) centre (-0.5, 14.8942) ccw
  line L17 (3.5, 26.3942) -> (3.5, 14.8942)
  arc A14 (3.5, 26.3942) -> (-0.5, 30.3942) centre (-0.5, 26.3942) ccw
  line L18 (-44, 30.3942) -> (-0.5, 30.3942)
  arc A15 (-44, 30.3942) -> (-48, 26.3942) centre (-44, 26.3942) ccw
  line L19 (-48, 14.8942) -> (-48, 26.3942)
  dimension "d421" = -3
extrude "Extrude69" add sketch "Sketch18" against normal blind 0.2 separate body contours A12 L16 A13 L17 A14 L18 A15 L19 makes body 23
extrude "Extrude70" cut sketch "Sketch18" against normal blind 0.2 contours A12 L16 A13 L17 A14 L18 A15 L19 bodies 15
move_body "Move1" bodies 6 to x (1, 0, 0) y (0, 1, 0) z (0, 0, 1) at (-1, 0, 0)
hidden bodies 1 2 3 4 5 6 7 8 9 10 11 12 13 14 15 16 19 20 21 22 23
named bodies: "Bodemplaat boven", "Body boven", "scherm bezel boven", "dmd bezel", "iphone", "display oled", "knop boven", "knop onder", "flipper rechts", "floipper links", "Top plaat boven", "Body onder", "Bodemplaat onder", "scherm bezel onder", "Top plaat onder", "ESPholder", "Button insert", "SideButton Holder", "USB-C Connector mount", "USB-C Connector mount (1)", "dmdFrame"
